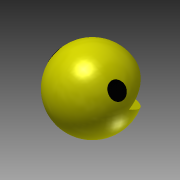
# Autodesk Inventor part: Pacman1
Saved by Autodesk Inventor 2015 (Build 190159000, 159)
## iProperties
Created: 2015-04-11
Part Number: Pacman1
Material: Generic
Document SubType Name: Modeling
Designer: tquinn
Density: 1 g/cm^3
Appearance: Default
Author: tquinn
Autodesk Inventor part; units mm, degrees
note: some values were not read from the file. Chosen so that the rebuilt part matches the saved one: direction of "Emboss1".
ref_plane "YZ Plane" through (0, 0, 0) normal (1, 0, 0) x (0, 1, 0)
sketch "Sketch1" plane through (0, 0, 0) normal (0, 1, 0) x (-1, 0, 0)
  circle A0 centre (0, 0) radius 500
  line L0 (0, 0) -> (0, -500)
  line L1 (0, 0) -> (0, 500)
  dimension "d0" = 1000
  constraints: 4 end point, 2 point on circle, 1 centre point, 1 coincident, 1 point on line, 1 vertical
  measures "d0" diameter of A0
revolve "Revolution1" add sketch "Sketch1" angle 360 about axis through (0, 0, 0) along (0, 0, 1) picked at (333.0045, -10.4651) contours A0 L0 L1
sketch "Sketch2" plane through (0, 0, 0) normal (1, 0, 0) x (0, 1, 0)
  circle A0 centre (0, 0) radius 500 projected
  line L0 (0, 0) -> (250, -433.0127)
  line L1 (0, 0) -> (500, 0) construction
  line L2 (0, 0) -> (-250, -433.0127)
  line L3 (0, 0) -> (500, 0) construction
  arc A1 (-250, -433.0127) -> (250, -433.0127) centre (0, 0) ccw
  dimension "d2" = 60
  dimension "d3" = 120
  constraints: 8 end point, 4 point on circle, 2 equal length, 2 horizontal, 1 centre point, 1 concentric
  measures "d2" angle of L0 L1
  measures "d3" angle of L2 L3
extrude "Extrusion1" cut sketch "Sketch2" along normal mid plane 1000 contours L2 L0 A0 picked at (-81.266, -323.1123)
ref_plane "Work Plane1" through (0, 433.0127, 250) normal (0, -0.8660254, -0.5) x (1, 0, 0)
sketch "Sketch3" plane through (0, 433.0127, 250) normal (0, -0.8660254, -0.5) x (1, 0, 0)
  arc A0 (-500, 0) -> (500, 0) centre (0, 0) ccw projected
  ellipse E0 centre (0, 0) end of major axis (-500, 0) minor radius 250 (-500, 0) -> (500, 0) ccw projected
  line L0 (500, 0) -> (500, 585.3972)
  circle A1 centre (0, 0) radius 500 projected
  constraints: 2 end point, 1 tangent, 1 vertical, 1 other
ref_plane "Work Plane2" through (500, 433.0127, 250) normal (1, 0, 0) x (0, 1, 0)
sketch "Sketch4" plane through (500, 433.0127, 250) normal (1, 0, 0) x (0, 1, 0)
  circle A0 centre (-203.3951, -164.3942) radius 100
  point P0 (-433.0127, -250)
  dimension "d6" = 200
  constraints: 1 centre point
  measures "d6" diameter of A0
emboss "Emboss1" sketch "Sketch4" operation add depth 2.54 direction (-1, 0, 0)
ref_plane "Work Plane4" through (0, 0, 0) normal (1, 0, 0) x (0, 1, 0)
ref_plane "Work Plane3" through (-500, 0, 0) normal (1, 0, 0) x (0, 1, 0)
mirror "Mirror1" about plane through (0, 0, 0) normal (1, 0, 0) of "Emboss1"
body "Solid1"
